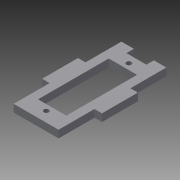
# Autodesk Inventor part: AngleTop
Saved by Autodesk Inventor 2013 (Build 170138000, 138)
## iProperties
Created: 2013-04-21
Part Number: AngleTop
Material: Generic
Document SubType Name: Modeling
Designer: fuji
Density: 1 g/cm^3
Author: fuji
Autodesk Inventor part; units mm, degrees
ref_plane "YZ Plane" through (0, 0, 0) normal (1, 0, 0) x (0, 1, 0)
ref_plane "XZ Plane" through (0, 0, 0) normal (0, 1, 0) x (-1, 0, 0)
ref_plane "XY Plane" through (0, 0, 0) normal (0, 0, 1) x (1, 0, 0)
sketch "Sketch1" plane through (0, 0, 0) normal (0, 1, 0) x (-1, 0, 0)
  line L0 (0, 0) -> (-19.05, 0)
  line L1 (-19.05, 0) -> (-19.05, -45.72)
  line L2 (-19.05, -45.72) -> (0, -45.72)
  line L3 (0, -45.72) -> (0, 0)
  line L4 (-19.05, -15.24) -> (-22.225, -15.24)
  line L5 (-22.225, -15.24) -> (-22.225, -30.48)
  line L6 (-22.225, -30.48) -> (-19.05, -30.48)
  line L7 (-19.05, -30.48) -> (-19.05, -15.24)
  line L8 (0, -30.48) -> (3.175, -30.48)
  line L9 (3.175, -30.48) -> (3.175, -15.24)
  line L10 (3.175, -15.24) -> (0, -15.24)
  line L11 (0, -15.24) -> (0, -30.48)
  dimension "d0" = 19.05
  dimension "d1" = 45.72
  dimension "d2" = 3.175
  dimension "d3" = 15.24
  dimension "d4" = 3.175
  dimension "d5" = 15.24
  dimension "d6" = 15.24
  constraints: 24 end point, 6 parallel, 3 horizontal, 3 perpendicular, 2 point on line, 1 collinear
  measures "d0" distance of L2.end L1.end
  measures "d1" distance of L1.end L0.end
  measures "d2" distance of L6.end L5.end
  measures "d3" distance of L5.end L4.end
  measures "d4" distance of L10.end L9.end
  measures "d5" distance of L9.end L8.end
  measures "d6" distance from line of L0 L4.end
extrude "Extrusion1" add sketch "Sketch1" along normal blind 3.175
sketch "Sketch2" plane through (0, 3.175, 0) normal (0, 1, 0) x (1, 0, 0)
  line L0 (-3.175, 30.48) -> (-3.175, 15.24) projected
  line L1 (19.05, 45.72) -> (0, 45.72) projected
  line L2 (5.2917, 45.72) -> (13.7583, 45.72)
  line L3 (13.7583, 45.72) -> (13.7583, 42.545)
  line L4 (13.7583, 42.545) -> (5.2917, 42.545)
  line L5 (5.2917, 42.545) -> (5.2917, 45.72)
  dimension "d9" = 8.4667
  dimension "d10" = 3.175
  dimension "d11" = 8.4667
  constraints: 8 end point, 2 parallel, 1 horizontal, 1 perpendicular, 1 point on line
  measures "d9" distance of L3.end L4.end
  measures "d10" distance of L2.end L3.end
  measures "d11" distance between parallel lines of L0 L5
extrude "Extrusion2" cut sketch "Sketch2" against normal blind 3.175
sketch "Sketch3" plane through (0, 3.175, 0) normal (0, 1, 0) x (1, 0, 0)
  line L0 (-3.175, 30.48) -> (-3.175, 15.24) projected
  line L1 (19.05, 45.72) -> (13.7583, 45.72) projected
  line L2 (3.525, 36.83) -> (15.525, 36.83)
  line L3 (15.525, 36.83) -> (15.525, 6.83)
  line L4 (15.525, 6.83) -> (3.525, 6.83)
  line L5 (3.525, 6.83) -> (3.525, 36.83)
  circle A0 centre (9.525, 4.33) radius 1.0541
  circle A1 centre (9.525, 39.33) radius 1.0541
  dimension "d14" = 12
  dimension "d15" = 30
  dimension "d16" = 6.7
  dimension "d17" = 8.89
  dimension "d18" = 2.1082
  dimension "d19" = 2.5
  dimension "d20" = 2.1082
  dimension "d21" = 2.5
  dimension "d22" = 6
  dimension "d23" = 6
  constraints: 8 end point, 2 centre point, 2 parallel, 1 horizontal, 1 perpendicular
  measures "d14" distance of L3.end L4.end
  measures "d15" distance of L2.end L3.end
  measures "d16" distance between parallel lines of L0 L5
  measures "d17" distance between parallel lines of L2 L1
  measures "d18" diameter of A0
  measures "d19" distance from line of A0.centre L4
  measures "d20" diameter of A1
  measures "d21" distance from line of A1.centre L2
  measures "d22" distance from line of L5 A1.centre
  measures "d23" distance from line of L5 A0.centre
extrude "Extrusion3" cut sketch "Sketch3" against normal blind 3.175
equation "\"d0\" = angleDepth - 2 * thick"
equation "\"d1\" = angleLength"
equation "\"d2\" = thick"
equation "\"d3\" = 0.333333 * angleLength"
equation "\"d4\" = thick"
equation "\"d5\" = 0.333333 * angleLength"
equation "\"d6\" = 0.333333 * angleLength"
equation "\"d7\" = thick"
equation "\"d9\" = 0.333333 * angleDepth"
equation "\"d10\" = thick"
equation "\"d11\" = 0.333333 * angleDepth"
equation "\"d12\" = thick"
equation "\"d14\" = servoWidth"
equation "\"d15\" = servoLength"
equation "\"d16\" = -0.5 * servoWidth + 0.5 * angleDepth"
equation "\"d17\" = servoOff"
equation "\"d18\" = servoHole"
equation "\"d19\" = -0.5 * servoLength + 0.5 * servoDist"
equation "\"d20\" = servoHole"
equation "\"d21\" = -0.5 * servoLength + 0.5 * servoDist"
equation "\"d22\" = 0.5 * servoWidth"
equation "\"d23\" = 0.5 * servoWidth"
equation "\"d24\" = thick"
equation "\"angleDepth\" = 25.4"
equation "\"thick\" = 3.175"
equation "\"angleLength\" = 45.72"
equation "\"servoLength\" = 30"
equation "\"servoWidth\" = 12"
equation "\"servoDist\" = 35"
equation "\"servoOff\" = 8.89"
equation "\"servoHole\" = 2.1082"
body "Solid1"
